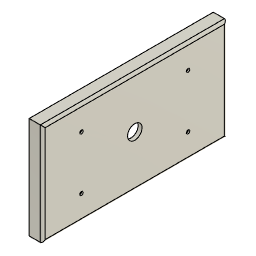
Bott_v2 (Autodesk Fusion 360 archive; units mm, degrees)
design "Bott_lid"
Autodesk Fusion 360 part; units mm, degrees
sketch "Sketch1" plane through (0, 0, 0) normal (1, 0, 0) x (0, 1, 0)
  line L0 (-95, 52.5) -> (95, 52.5)
  line L1 (95, 52.5) -> (95, -52.5)
  line L2 (95, -52.5) -> (-95, -52.5)
  line L3 (-95, -52.5) -> (-95, 52.5)
  line L4 (95, 52.5) -> (-95, -52.5) construction
  line L5 (-95, 52.5) -> (95, -52.5) construction
  line L6 (92, -49.5) -> (-92, -49.5)
  line L7 (-92, -49.5) -> (-92, 49.5)
  line L8 (-92, 49.5) -> (92, 49.5)
  line L9 (92, 49.5) -> (92, -49.5)
  dimension "d1" = 190
  dimension "d2" = 105
  dimension "d5" = 3
  constraint horizontal L0
  constraint vertical L1
  constraint horizontal L2
  constraint vertical L3
  constraint midpoint origin L4
  measures "d1" distance of L0.start L0.end
  measures "d2" distance of L0.start L2.end
extrude "Extrude1" add sketch "Sketch1" along normal blind 14 contours L0 L1 L2 L3 | L6 L7 L8 L9
extrude "Extrude2" cut sketch "Sketch1" along normal blind 10 contours L6 L7 L8 L9
fillet "Fillet1" radius 2.5 4 edges at (14, 0, -52.5) (14, 95, 0) (14, 0, 52.5) (14, -95, 0)
sketch "Sketch2" plane through (14, 0, 0) normal (1, 0, 0) x (0, 1, 0)
  line L0 (92.5, 50) -> (-92.5, 50)
  line L1 (-92.5, 50) -> (-92.5, -50)
  line L2 (-92.5, -50) -> (92.5, -50)
  line L3 (92.5, -50) -> (92.5, 50)
  circle A0 centre (0, 0) radius 7.5
  dimension "d10" = 15
  constraint coincident A0.centre origin
  measures "d10" diameter of A0
extrude "Extrude3" cut sketch "Sketch2" against normal blind 40 contours A0
sketch "Sketch3" plane through (14, 0, 0) normal (1, 0, 0) x (0, 1, 0)
  circle A0 centre (0, 0) radius 7.5
  line L0 (92.5, 50) -> (-92.5, 50)
  line L1 (-92.5, 50) -> (-92.5, -50)
  line L2 (-92.5, -50) -> (92.5, -50)
  line L3 (92.5, -50) -> (92.5, 50)
  line L4 (-55, 27.5) -> (55, 27.5)
  line L5 (55, 27.5) -> (55, -27.5)
  line L6 (55, -27.5) -> (-55, -27.5)
  line L7 (-55, -27.5) -> (-55, 27.5)
  line L8 (55, 27.5) -> (-55, -27.5) construction
  line L9 (-55, 27.5) -> (55, -27.5) construction
  dimension "d13" = 110
  dimension "d14" = 55
  constraint horizontal L4
  constraint vertical L5
  constraint horizontal L6
  constraint vertical L7
  constraint midpoint A0.centre L9
  measures "d13" distance of L4.start L4.end
  measures "d14" distance of L4.start L6.end
hole "Hole1" at (14, 55, 27.5) at (14, -55, 27.5) at (14, -55, -27.5) at (14, 55, -27.5) direction (-1, 0, 0) diameter 1.371 depth 10 tip angle 118 counterbore diameter 3.5 counterbore depth 1.6
thread "Thread1" "ISO Metric profile 1.7 M1.7x0.35 6H"
